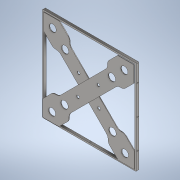
# Autodesk Inventor part: Chassis
Saved by Autodesk Inventor 2020.3 (Build 243373000, 373)
## iProperties
Created: 2022-07-02
Part Number: Chassis
Material: Generic
Document SubType Name: Modeling
Designer: karimi2
Density: 1 g/cm^3
Appearance: Steel - Polished
Author: karimi2
Autodesk Inventor part; units mm, degrees
ref_plane "YZ Plane" through (0, 0, 0) normal (1, 0, 0) x (0, 1, 0)
ref_plane "XZ Plane" through (0, 0, 0) normal (0, 1, 0) x (-1, 0, 0)
ref_plane "XY Plane" through (0, 0, 0) normal (0, 0, 1) x (1, 0, 0)
sketch "Sketch1" plane through (0, 0, 0) normal (0, 0, 1) x (1, 0, 0)
  line L0 (0, 1487) -> (0, 5) construction
  line L1 (0, 0) -> (160, 0)
  line L2 (160, 0) -> (160, 320)
  line L3 (160, 320) -> (0, 320)
  line L4 (0, 0) -> (5, 0)
  line L5 (0, 0) -> (0, 5)
  line L6 (0, 5) -> (155, 5)
  line L7 (155, 5) -> (155, 315)
  line L8 (155, 315) -> (0, 315)
  line L9 (0, 0) -> (-160, 0)
  line L10 (-160, 0) -> (-160, 320)
  line L11 (-160, 320) -> (0, 320)
  line L12 (0, 5) -> (-155, 5)
  line L13 (-155, 5) -> (-155, 315)
  line L14 (-155, 315) -> (0, 315)
  dimension "d12" = 160
  dimension "d13" = 320
  dimension "d14" = 5
  dimension "d15" = 5
  dimension "d19" = 310
  dimension "d20" = 155
  dimension "d21" = 1487
  constraints: 30 end point, 4 perpendicular, 4 symmetric about line, 3 point on line, 2 parallel, 1 horizontal, 1 vertical
  measures "d12" distance of L1.start L1.end
  measures "d13" distance of L1.end L2.end
  measures "d14" distance of L1.start L4.end
  measures "d15" distance of L0.end L1.start
  measures "d19" distance of L6.end L7.end
  measures "d20" distance of L0.end L6.end
  measures "d21" distance from line of L0.start L1
extrude "Extrusion2" add sketch "Sketch1" along normal mid plane 8
fillet "Fillet2" radius 2 4 edges at (160, 320, 0) (-160, 320, 0) (160, 0, 0) (-160, 0, 0)
ref_plane "Work Plane1" through (0, 0, 4) normal (0, 0, 1) x (1, 0, 0)
sketch "Sketch2" plane through (0, 0, 4) normal (0, 0, 1) x (1, 0, 0)
  line L0 (-155, 315) -> (155, 5)
  line L1 (-137.5, 332.5) -> (172.5, 22.5)
  line L2 (-173, 297) -> (137, -13)
  line L3 (-173, 297) -> (-137.5, 332.5)
  circle A0 centre (-123.1802, 283.1802) radius 12
  circle A1 centre (-80.7538, 240.7538) radius 12.5
  line L4 (137, -13) -> (172.5, 22.5)
  circle A2 centre (123.1802, 36.8198) radius 12
  circle A3 centre (80.7538, 79.2462) radius 12.5
  circle A4 centre (34.7918, 125.2082) radius 5
  circle A5 centre (-34.7918, 194.7918) radius 5
  line L5 (-155, 315) -> (-155, 5) projected
  line L6 (-155, 315) -> (-155, 260)
  line L7 (-155, 260) -> (-120, 225)
  line L8 (-155, 315) -> (-100, 315)
  line L9 (-155, 315) -> (155, 315) projected
  line L10 (-100, 315) -> (-65, 280)
  line L11 (155, 5) -> (-155, 5) projected
  line L12 (155, 5) -> (100, 5)
  line L13 (155, 5) -> (155, 60)
  line L14 (155, 315) -> (155, 5) projected
  line L15 (-65, 280) -> (-68.2954, 239.7342)
  line L16 (-120, 225) -> (-79.7342, 228.2954)
  line L17 (155, 60) -> (120, 95)
  line L18 (100, 5) -> (65, 40)
  line L19 (65, 40) -> (68.2954, 80.2658)
  line L20 (120, 95) -> (79.7342, 91.7046)
  line L21 (155, 60) -> (182.5, 32.5)
  line L22 (182.5, 32.5) -> (172.5, 22.5)
  line L23 (100, 5) -> (127.5, -22.5)
  line L24 (127.5, -22.5) -> (137, -13)
  line L25 (-100, 315) -> (-127.5, 342.5)
  line L26 (-127.5, 342.5) -> (-137.5, 332.5)
  line L27 (-173, 297) -> (-182.5, 287.5)
  line L28 (-182.5, 287.5) -> (-155, 260)
  point P0 (0, 0)
  point P1 (66.4374, 57.5626)
  point P2 (119, 5)
  point P3 (101.513, 93.487)
  point P4 (155, 40)
  point P5 (-66.513, 261.513)
  point P6 (-120, 315)
  point P7 (-102.4374, 226.4374)
  point P8 (-155, 279)
  dimension "d30" = 24.7487
  dimension "d31" = 25.4558
  dimension "d32" = 50.2046
  dimension "d33" = 24
  dimension "d34" = 25
  dimension "d35" = 45
  dimension "d36" = 105
  dimension "d37" = 24
  dimension "d38" = 25
  dimension "d39" = 45
  dimension "d40" = 35.5
  dimension "d41" = 105
  dimension "d42" = 438.4062
  dimension "d43" = 0
  dimension "d44" = 0
  dimension "d45" = 10
  dimension "d46" = 10
  dimension "d47" = 170
  dimension "d48" = 170
  dimension "d111" = 55
  dimension "d112" = 55
  dimension "d114" = 45
  dimension "d115" = 45
  dimension "d116" = 55
  dimension "d117" = 55
  dimension "d118" = 35
  dimension "d119" = 35
  dimension "d121" = 45
  dimension "d122" = 45
  dimension "d123" = 35
  dimension "d124" = 35
  constraints: 50 end point, 12 point on line, 6 centre point, 4 parallel, 4 point on circle, 4 tangent, 3 perpendicular
  measures "d30" distance between parallel lines of L0 L1
  measures "d31" distance between parallel lines of L0 L2
  measures "d32" distance of L2.start L1.start
  measures "d33" diameter of A0
  measures "d34" diameter of A1
  measures "d35" distance from line of A0.centre L3
  measures "d36" distance from line of A1.centre L3
  measures "d37" diameter of A2
  measures "d38" diameter of A3
  measures "d39" distance from line of A2.centre L4
  measures "d40" horizontal distance of L2.end L1.end
  measures "d41" distance from line of A3.centre L4
  measures "d42" distance between parallel lines of L4 L3
  measures "d43" distance from line of L0.end L4
  measures "d44" distance from line of L4.end L1
  measures "d45" diameter of A4
  measures "d46" diameter of A5
  measures "d47" distance from line of A4.centre L4
  measures "d48" distance from line of A5.centre L3
  measures "d111" distance of L0.start L6.end
  measures "d112" distance of L0.start L8.end
  measures "d114" angle of L10 L9
  measures "d115" angle of L5 L7
  measures "d116" distance of L0.end L12.end
  measures "d117" distance of L0.end L13.end
  measures "d118" horizontal distance of L6.end L7.end
  measures "d119" horizontal distance of L8.end L10.end
  measures "d121" angle of L11 L18
  measures "d122" angle of L14 L17
  measures "d123" horizontal distance of L13.end L17.end
  measures "d124" horizontal distance of L12.end L18.end
extrude "Extrusion3" add sketch "Sketch2" along normal blind 2 contours L8 L1 L15 A1 L0 A0 | L0 A0 A1 L16 L2 L5 | L2 L16 L7 L5 | L8 L10 L15 L1 | L16 A1 L0 A5 A4 A3 L19 L2 | L1 L20 A3 L0 A4 A5 A1 L15 | L19 A3 L0 A2 L11 L2 | L2 L11 L18 L19 | L20 L17 L13 L1 | L1 L13 L0 A2 A3 L20
ref_plane "Work Plane2" through (0, 0, 6) normal (0, 0, 1) x (1, 0, 0)
sketch "Sketch3" plane through (0, 0, 6) normal (0, 0, 1) x (1, 0, 0)
  line L0 (-155, 5) -> (155, 315)
  line L1 (-172.5, 22.5) -> (137.5, 332.5)
  line L2 (-137.5, -12.5) -> (172.5, 297.5)
  line L3 (-172.5, 22.5) -> (-137.5, -12.5)
  line L4 (137.5, 332.5) -> (172.5, 297.5)
  circle A0 centre (123.1802, 283.1802) radius 12
  circle A1 centre (80.7538, 240.7538) radius 12.5
  circle A2 centre (34.7918, 194.7918) radius 5
  circle A3 centre (-34.7918, 125.2082) radius 5
  circle A4 centre (-80.7538, 79.2462) radius 12.5
  circle A5 centre (-123.1802, 36.8198) radius 12
  line L5 (155, 315) -> (155, 60) projected
  line L6 (155, 315) -> (100, 315)
  line L7 (155, 315) -> (-155, 315) projected
  line L8 (100, 315) -> (65, 280)
  line L9 (65, 280) -> (68.2954, 239.7342)
  line L10 (155, 315) -> (155, 260)
  line L11 (155, 260) -> (120, 225)
  line L12 (120, 225) -> (79.7342, 228.2954)
  line L13 (-155, 5) -> (-155, 260) projected
  line L14 (-155, 5) -> (-155, 60)
  line L15 (-155, 60) -> (-120, 95)
  line L16 (100, 5) -> (-155, 5) projected
  line L17 (-155, 5) -> (-100, 5)
  line L18 (-100, 5) -> (-65, 40)
  line L19 (-65, 40) -> (-68.2954, 80.2658)
  line L20 (-120, 95) -> (-79.7342, 91.7046)
  point P0 (0, 0)
  point P1 (-68.2538, 79.2462)
  point P2 (66.513, 261.513)
  point P3 (-101.513, 93.487)
  point P4 (-66.513, 58.487)
  point P5 (101.513, 226.513)
  dimension "d55" = 24.7487
  dimension "d56" = 24.7487
  dimension "d57" = 24
  dimension "d58" = 25
  dimension "d59" = 10
  dimension "d60" = 45
  dimension "d61" = 35
  dimension "d62" = 105
  dimension "d63" = 170
  dimension "d64" = 45
  dimension "d65" = 105
  dimension "d66" = 170
  dimension "d67" = 438.4062
  dimension "d68" = 0
  dimension "d69" = 438.4062
  dimension "d125" = 55
  dimension "d126" = 55
  dimension "d127" = 45
  dimension "d128" = 35
  dimension "d129" = 45
  dimension "d130" = 35
  dimension "d131" = 55
  dimension "d132" = 55
  dimension "d133" = 45
  dimension "d134" = 35
  dimension "d135" = 45
  dimension "d136" = 35
  constraints: 34 end point, 10 point on line, 6 centre point, 5 point on circle, 3 equal radius, 3 parallel, 2 tangent, 1 perpendicular
  measures "d55" distance between parallel lines of L0 L1
  measures "d56" distance between parallel lines of L0 L2
  measures "d57" diameter of A0
  measures "d58" diameter of A1
  measures "d59" diameter of A2
  measures "d60" distance from line of A0.centre L4
  measures "d61" horizontal distance of L2.end L1.end
  measures "d62" distance from line of A1.centre L4
  measures "d63" distance from line of A2.centre L4
  measures "d64" distance from line of A5.centre L3
  measures "d65" distance from line of A4.centre L3
  measures "d66" distance from line of A3.centre L3
  measures "d67" distance between parallel lines of L3 L4
  measures "d68" distance from line of L0.end L4
  measures "d69" distance from line of L0.start L4
  measures "d125" distance of L0.end L6.end
  measures "d126" distance of L0.end L10.end
  measures "d127" angle of L7 L8
  measures "d128" horizontal distance of L6.end L8.end
  measures "d129" angle of L5 L11
  measures "d130" horizontal distance of L10.end L11.end
  measures "d131" distance of L0.start L14.end
  measures "d132" distance of L0.start L17.end
  measures "d133" angle of L16 L18
  measures "d134" horizontal distance of L17.end L18.end
  measures "d135" angle of L13 L15
  measures "d136" horizontal distance of L14.end L15.end
extrude "Extrusion4" add sketch "Sketch3" along normal blind 2 contours L13 L1 L20 A4 L0 A5 | L0 A5 A4 L19 L2 L16 | L13 L15 L20 L1 | L2 L19 L18 L16 | L1 L9 A1 L0 A2 A3 A4 L20 | L19 A4 L0 A3 A2 A1 L12 L2 | L9 L8 L6 L1 | L1 L6 L0 A0 A1 L9 | L12 A1 L0 A0 L5 L2 | L2 L5 L11 L12
ref_plane "Work Plane4" through (160, 2, -4) normal (1, 0, 0) x (0, 0, -1)
sketch "Sketch5" plane through (160, 2, -4) normal (1, 0, 0) x (0, 0, -1)
  circle A0 centre (-4, 158) radius 2
  circle A1 centre (-4, 58) radius 2
  circle A2 centre (-4, 258) radius 2
  line L0 (0, 318) -> (-8, 318) projected
  point P0 (-4, -2)
  dimension "d84" = 4
  dimension "d85" = 4
  dimension "d86" = 4
  dimension "d87" = 60
  dimension "d88" = 100
  dimension "d89" = 100
  dimension "d90" = 60
  constraints: 3 centre point, 2 vertical alignment
  measures "d84" diameter of A0
  measures "d85" diameter of A1
  measures "d86" diameter of A2
  measures "d87" distance of A1.centre point (-4, -2)
  measures "d88" distance of A0.centre A1.centre
  measures "d89" distance of A2.centre A0.centre
  measures "d90" distance from line of L0 A2.centre
extrude "Extrusion6" cut sketch "Sketch5" against normal blind 8
ref_plane "Work Plane6" through (-158, 0, -4) normal (0, -1, 0) x (1, 0, 0)
sketch "Sketch7" plane through (-158, 0, -4) normal (0, -1, 0) x (1, 0, 0)
  circle A0 centre (158, 4) radius 2
  circle A1 centre (258, 4) radius 2
  circle A2 centre (58, 4) radius 2
  dimension "d104" = 4
  dimension "d105" = 4
  dimension "d106" = 4
  dimension "d107" = 100
  dimension "d108" = 100
  constraints: 3 centre point, 2 horizontal alignment, 1 coincident
  measures "d104" diameter of A0
  measures "d105" diameter of A1
  measures "d106" diameter of A2
  measures "d107" distance of A1.centre point (158, 4)
  measures "d108" distance of A2.centre point (158, 4)
extrude "Extrusion8" cut sketch "Sketch7" against normal blind 8
fillet "Fillet3" radius 20 16 edges at (65, 40, 5) (66.4374, 57.5626, 5) (120, 95, 5) (101.513, 93.487, 5) (66.513, 261.513, 7) (65, 280, 7) (-120, 225, 5) (-102.4374, 226.4374, 5) (-101.513, 93.487, 7) (-120, 95, 7) (-66.513, 58.487, 7) (-65, 40, 7) (101.513, 226.513, 7) (120, 225, 7) (-65, 280, 5) (-66.513, 261.513, 5)
body "Solid2"
